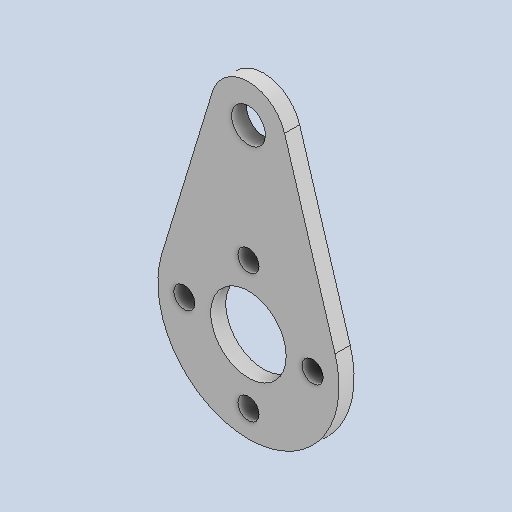
# Autodesk Inventor part: lever
Saved by Autodesk Inventor 2022 (Build 260153000, 153)
## iProperties
Created: 2022-10-18
Part Number: lever
Material: 一般
Document SubType Name: Modeling
Designer: haya
Density: 1 g/cm^3
Appearance: 既定
Author: haya
Autodesk Inventor part; units mm, degrees
ref_plane "YZ Plane" through (0, 0, 0) normal (1, 0, 0) x (0, 1, 0)
ref_plane "XZ Plane" through (0, 0, 0) normal (0, 1, 0) x (-1, 0, 0)
ref_plane "XY Plane" through (0, 0, 0) normal (0, 0, 1) x (1, 0, 0)
sketch "スケッチ1" plane through (0, 0, 0) normal (0, 0, 1) x (1, 0, 0)
  circle A0 centre (0, 0) radius 5
  arc A1 (-11.4782, 3.5) -> (11.4782, 3.5) centre (0, 0) ccw
  arc A2 (4.7826, 25.4583) -> (-4.7826, 25.4583) centre (0, 24) ccw
  line L0 (-4.7826, 25.4583) -> (-11.4782, 3.5)
  line L1 (4.7826, 25.4583) -> (11.4782, 3.5)
  dimension "d0" = 10
  dimension "d1" = 24
  dimension "d2" = 10
  dimension "d3" = 24
  constraints: 4 end point, 4 point on circle, 4 tangent, 3 centre point, 2 coincident, 1 vertical alignment
  measures "d0" diameter of A0
  measures "d1" diameter of A1
  measures "d2" diameter of A2
  measures "d3" distance of point (0, 0) A2.centre
extrude "押し出し1" add sketch "スケッチ1" along normal blind 2
sketch "スケッチ2" plane through (0, 0, 2) normal (0, 0, 1) x (1, 0, 0)
  line L0 (0, 0) -> (12, 0) construction
  arc A0 (-11.4782, 3.5) -> (11.4782, 3.5) centre (0, 0) ccw projected
  line L1 (0, 0) -> (0, 12) construction
  line L2 (0, 0) -> (-12, 0) construction
  line L3 (0, 0) -> (0, -12) construction
  point P0 (8.5, 0)
  point P1 (0, 8.5)
  point P2 (-8.5, 0)
  point P3 (0, -8.5)
  dimension "d6" = 8.5
  dimension "d9" = 360
  constraints: 8 end point, 4 point on line, 2 coincident, 1 horizontal, 1 point on circle, 15 other
  measures "d6" distance of point (8.5, 0) L0.start
hole "穴1" at (8.5, 0, 2) at (0, 8.5, 2) at (-8.5, 0, 2) at (0, -8.5, 2) direction (0, 0, -1) diameter 2.8 end through all
sketch "スケッチ3" plane through (0, 0, 2) normal (0, 0, 1) x (1, 0, 0)
  arc A0 (4.7826, 25.4583) -> (-4.7826, 25.4583) centre (0, 24) ccw projected
  point P0 (0, 0)
hole "穴2" at (0, 24, 2) direction (0, 0, -1) diameter 4.5 end through all
